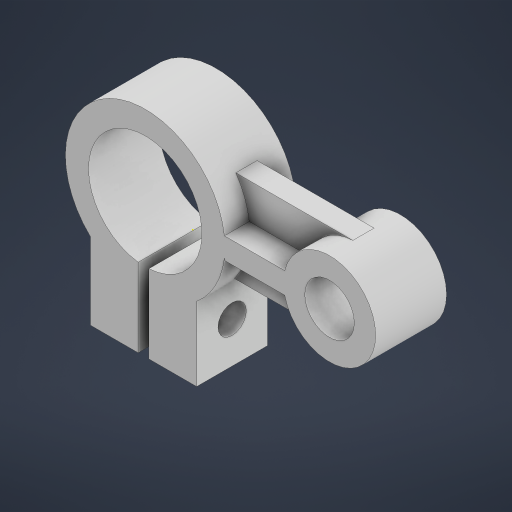
# Autodesk Inventor part: Część9
Saved by Autodesk Inventor 2023 (Build 270158000, 158)
## iProperties
Created: 2023-05-07
Part Number: Część9
Material: Ogólny
Document SubType Name: Modeling
Designer: Adam
Density: 1 g/cm^3
Appearance: Domyślna
Author: Adam
Autodesk Inventor part; units mm, degrees
ref_plane "YZ Plane" through (0, 0, 0) normal (1, 0, 0) x (0, 1, 0)
ref_plane "XZ Plane" through (0, 0, 0) normal (0, 1, 0) x (-1, 0, 0)
ref_plane "XY Plane" through (0, 0, 0) normal (0, 0, 1) x (1, 0, 0)
sketch "Szkic1" plane through (0, 0, 0) normal (0, 0, 1) x (1, 0, 0)
  circle A0 centre (-13.3747, 0.2773) radius 22.5
  circle A1 centre (38.6246, 0.0082) radius 13
  line L0 (8.9598, 3.0013) -> (25.9772, 3.0013)
  line L1 (25.9772, 3.0013) -> (25.9772, -2.9987)
  line L2 (25.9772, -2.9987) -> (8.9598, -2.9987)
  line L3 (8.9598, -2.9987) -> (8.9598, 3.0013)
  line L4 (25.9772, 3.0013) -> (8.9598, -2.9987) construction
  line L5 (1.1462, -22.2227) -> (1.1462, -37.7227)
  line L6 (1.1462, -37.7227) -> (-28.8538, -37.7227)
  line L7 (-28.8538, -37.7227) -> (-28.8538, -22.2227)
  line L8 (-28.8538, -22.2227) -> (-28.8538, -16.052)
  line L9 (1.1462, -22.2227) -> (1.1462, -16.9097)
  point P0 (0, 0)
  point P1 (17.4685, 0.0013)
  point P2 (-13.8538, -22.2176)
  point P3 (8.9598, -2.4467)
  point P4 (25.9739, 3.0013)
  dimension "d1" = 26
  dimension "d0" = 45
  dimension "d2" = 52
  dimension "d3" = 6
  dimension "d4" = 30
  dimension "d5" = 38
  constraints: 20 end point, 4 parallel, 4 point on circle, 1 centre point, 1 horizontal, 1 midpoint, 1 perpendicular, 1 vertical, 3 other
  measures "d0" diameter of A0
  measures "d2" distance of point (38.625, 0.008) A0.centre
  measures "d3" distance of L0.end L1.end
  measures "d4" distance of L5.end L6.end
  measures "d5" distance from line of A0.centre L6
extrude "Wyciągnięcie proste1" add sketch "Szkic1" along normal mid plane 20
sketch "Szkic2" plane through (0, 0, 10) normal (0, 0, 1) x (1, 0, 0)
  point P0 (0, 0)
sketch "Szkic3" plane through (8.9598, 3.0013, 10) normal (0, 1, 0) x (1, 0, 0)
  line L0 (29.8394, 10) -> (-7.8136, 10)
  line L1 (-7.8136, 20) -> (-7.8136, 0) projected
  line L2 (-7.8136, 13) -> (29.8394, 13)
  line L3 (29.8394, 13) -> (29.8394, 7)
  line L4 (29.8394, 7) -> (-7.8136, 7)
  line L5 (-7.8136, 7) -> (-7.8136, 13)
  line L6 (-7.8136, 13) -> (29.8394, 7) construction
  line L7 (29.8394, 13) -> (-7.8136, 7) construction
  point P0 (-8.9598, 10)
  point P1 (11.0129, 10)
  dimension "d8" = 6
  constraints: 14 end point, 4 midpoint, 2 parallel, 1 horizontal, 1 perpendicular
  measures "d8" distance of L2.end L3.end
extrude "Wyciągnięcie proste2" add sketch "Szkic3" along normal blind 10 and the other way blind 16
sketch "Szkic4" plane through (0, 0, 10) normal (0, 0, 1) x (1, 0, 0)
  arc A0 (8.9598, 3.0013) -> (-28.8538, -16.052) centre (-13.3747, 0.2773) ccw projected
  arc A1 (25.9772, -2.9987) -> (25.9739, 3.0013) centre (38.6246, 0.0082) ccw projected
  point P0 (0, 0)
  constraints: 2 coincident
sketch "Szkic5" plane through (0, 0, 10) normal (0, 0, 1) x (1, 0, 0)
  line L0 (-12.3538, -38.025) -> (-15.3538, -38.025)
  line L1 (-15.3538, -38.025) -> (-15.3538, -14.6448)
  line L2 (-15.3538, -14.6448) -> (-12.3538, -14.6448)
  line L3 (-12.3538, -14.6448) -> (-12.3538, -38.025)
  line L4 (-12.3538, -38.025) -> (-15.3538, -14.6448) construction
  line L5 (-15.3538, -38.025) -> (-12.3538, -14.6448) construction
  point P0 (0, 0)
  point P1 (-13.8538, -26.3349)
  dimension "d13" = 3
  constraints: 12 end point, 2 midpoint, 2 parallel, 1 horizontal, 1 perpendicular
  measures "d13" distance of L1.end L2.end
hole "Otwór1" at (-13.3747, 0.2773, 10) direction (0, 0, -1) diameter 32 end through all
sketch "Szkic6" plane through (0, 0, 10) normal (0, 0, 1) x (1, 0, 0)
  arc A0 (25.9772, -2.9987) -> (25.9739, 3.0013) centre (38.6246, 0.0082) ccw projected
  point P0 (0, 0)
  constraints: 1 coincident
hole "Otwór2" at (38.6246, 0.0082, 10) direction (0, 0, -1) diameter 14 end through all
extrude "Wyciągnięcie proste3" cut sketch "Szkic5" against normal through all
sketch "Szkic7" plane through (1.1462, -37.7227, 10) normal (1, 0, 0) x (0, 0, -1)
  point P0 (10, 37.7227)
  point P1 (10, 11.5)
hole "Otwór3" at (1.1462, -26.2227, 0) direction (-1, 0, 0) diameter 8 end through all
